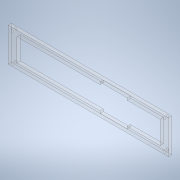
# Autodesk Inventor part: Template-Fixture-Top
Saved by Autodesk Inventor 2021 (Build 250183000, 183)
## iProperties
Created: 2020-06-16
Part Number: Template-Fixture-Top
Material: Polycarbonate, Clear
Document SubType Name: Modeling
Designer: lucas
Density: 1.2 g/cm^3
Appearance: Polycarbonate - Clear
Project: 4Wire-FDM
Author: lucas
Revision Number: RLS_004
Autodesk Inventor part; units mm, degrees
ref_plane "YZ Plane" through (0, 0, 0) normal (1, 0, 0) x (0, 1, 0)
ref_plane "XZ Plane" through (0, 0, 0) normal (0, 1, 0) x (-1, 0, 0)
ref_plane "XY Plane" through (0, 0, 0) normal (0, 0, 1) x (1, 0, 0)
sketch "Sketch1" plane through (0, 0, 0) normal (0, 0, 1) x (1, 0, 0)
  line L0 (93.3916, -12.6) -> (93.3916, 12.6)
  line L1 (53.9763, -12.6) -> (93.3916, -12.6)
  line L2 (53.9763, -15.2) -> (53.9763, -12.6)
  line L3 (38.2753, -15.2) -> (53.9763, -15.2)
  line L4 (38.2753, -15.2) -> (23.4296, -15.2)
  line L5 (23.4296, -12.6) -> (23.4296, -15.2)
  line L6 (-76.0546, -12.6) -> (23.4296, -12.6)
  line L7 (23.4296, 12.6) -> (-76.0546, 12.6)
  line L8 (23.4296, 15.2) -> (23.4296, 12.6)
  line L9 (-76.0546, 12.6) -> (-76.0546, -12.6)
  line L10 (23.4296, 15.2) -> (53.9763, 15.2)
  line L11 (53.9763, 15.2) -> (53.9763, 12.6)
  line L12 (53.9763, 12.6) -> (93.3916, 12.6)
  line L13 (-77.0546, 13.6) -> (22.4296, 13.6)
  line L14 (22.4296, 13.6) -> (22.4296, 16.2)
  line L15 (22.4296, 16.2) -> (54.9763, 16.2)
  line L16 (54.9763, 16.2) -> (54.9763, 13.6)
  line L17 (54.9763, 13.6) -> (94.3916, 13.6)
  line L18 (94.3916, 13.6) -> (94.3916, -13.6)
  line L19 (94.3916, -13.6) -> (54.9763, -13.6)
  line L20 (54.9763, -13.6) -> (54.9763, -16.2)
  line L21 (54.9763, -16.2) -> (38.2753, -16.2)
  line L22 (38.2753, -16.2) -> (22.4296, -16.2)
  line L23 (22.4296, -16.2) -> (22.4296, -13.6)
  line L24 (22.4296, -13.6) -> (-77.0546, -13.6)
  line L25 (-77.0546, -13.6) -> (-77.0546, 13.6)
  line L26 (22.4296, -16.2) -> (22.4296, -20.2) construction
  line L27 (22.4296, -20.2) -> (-87.5704, -20.2)
  line L28 (-87.5704, -20.2) -> (-87.5704, 20.2)
  line L29 (-87.5704, 20.2) -> (22.4296, 20.2)
  line L30 (104.4296, -20.2) -> (22.4296, -20.2)
  line L31 (22.4296, 20.2) -> (104.4296, 20.2)
  line L32 (104.4296, 20.2) -> (104.4296, -20.2)
  line L33 (-87.5704, 20.2) -> (-87.5704, 17.2)
  line L34 (-87.5704, 17.2) -> (-82.5704, 17.2) construction
  circle A0 centre (-82.5704, 17.2) radius 1.6
  line L35 (-87.5704, -20.2) -> (-87.5704, -17.2)
  line L36 (-87.5704, -17.2) -> (-82.5704, -17.2) construction
  circle A1 centre (-82.5704, -17.2) radius 1.6
  line L37 (104.4296, -20.2) -> (104.4296, -17.2) construction
  line L38 (104.4296, -17.2) -> (99.4296, -17.2) construction
  circle A2 centre (99.4296, -17.2) radius 1.6
  line L39 (104.4296, 20.2) -> (104.4296, 17.2) construction
  line L40 (104.4296, 17.2) -> (99.4296, 17.2) construction
  circle A3 centre (99.4296, 17.2) radius 1.6
  dimension "d0" = 1
  dimension "d1" = 4
  dimension "d2" = 110
  dimension "d3" = 40.4
  dimension "d5" = 82
  dimension "d8" = 3
  dimension "d9" = 5
  dimension "d10" = 3.2
  dimension "d11" = 3
  dimension "d12" = 5
  dimension "d13" = 3.2
  dimension "d14" = 3
  dimension "d15" = 5
  dimension "d16" = 3.2
  dimension "d17" = 3
  dimension "d18" = 5
  dimension "d19" = 3.2
  constraints: 82 end point, 11 perpendicular, 5 point on line, 4 centre point, 4 coincident, 2 horizontal, 1 parallel, 1 vertical, 12 other
  measures "d0" distance between parallel lines of L7 L13
  measures "d1" distance of L22.end L26.end
  measures "d2" distance of L26.end L27.end
  measures "d3" distance of L27.end L28.end
  measures "d5" distance of L29.end L31.end
  measures "d8" distance of L28.end L33.end
  measures "d9" distance of L33.end L34.end
  measures "d10" diameter of A0
  measures "d11" distance of L27.end L35.end
  measures "d12" distance of L35.end L36.end
  measures "d13" diameter of A1
  measures "d14" distance of L30.start L37.end
  measures "d15" distance of L37.end L38.end
  measures "d16" diameter of A2
  measures "d17" distance of L31.end L39.end
  measures "d18" distance of L39.end L40.end
  measures "d19" diameter of A3
extrude "Extrusion1" add sketch "Sketch1" against normal blind 4 contours L27 L28 L29 L31 L32 L30
body "Solid1"
